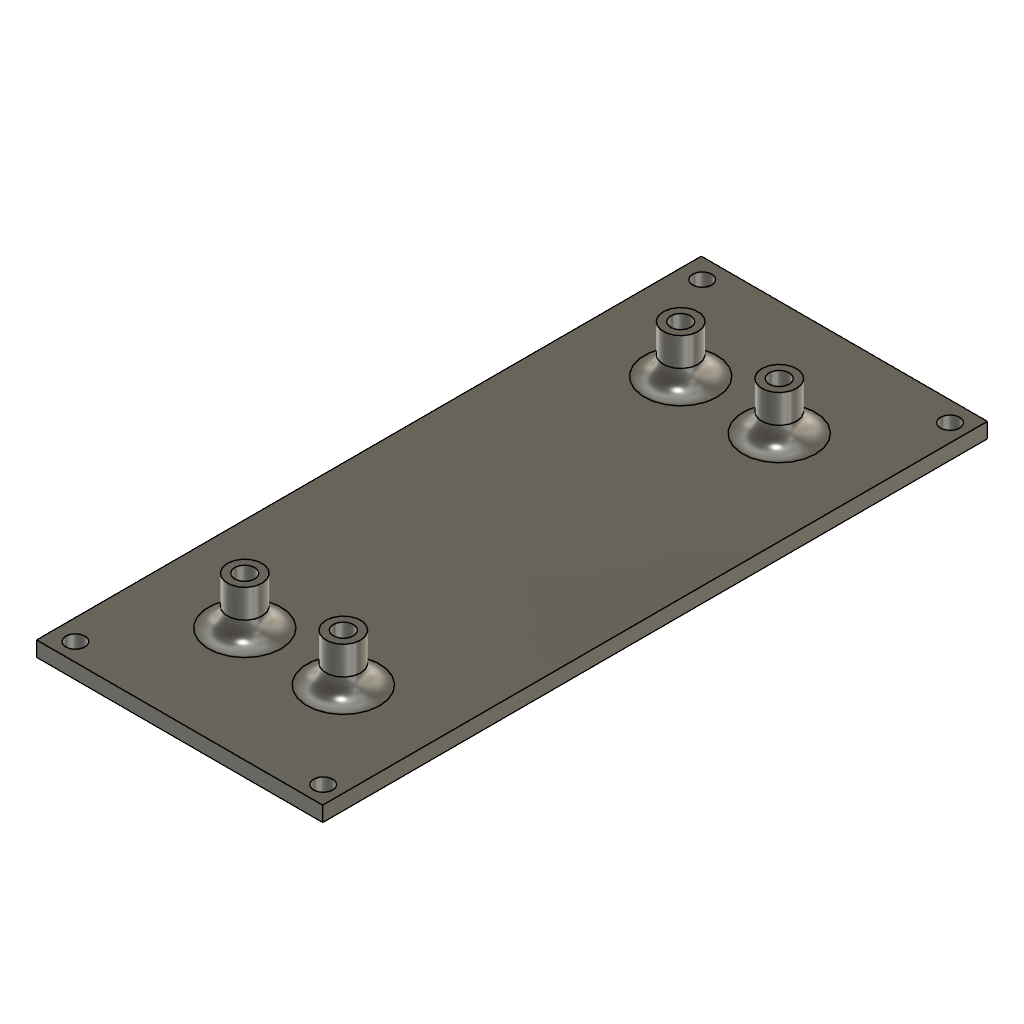
raspberry_pi_pico_mounting_board (Autodesk Fusion 360 design; units mm, degrees)
Autodesk Fusion 360 part; units mm, degrees
sketch "Sketch1" plane through (0, 0, 0) normal (0, 0, 1) x (1, 0, 0)
  line L0 (0, 0) -> (30.2, 0)
  line L1 (30.2, 0) -> (30.2, 70.15)
  line L2 (30.2, 70.15) -> (0, 70.15)
  line L3 (0, 70.15) -> (0, 0)
  dimension "d1" = 30.2
  dimension "d2" = 70.15
  constraint horizontal L0
  constraint vertical L1
  constraint horizontal L2
  constraint vertical L3
  constraint coincident L0.start L3.end
  measures "d1" distance of L0.start L0.end
  measures "d2" distance of L0.start L2.end
extrude "Extrude1" add sketch "Sketch1" along normal blind 1.6
sketch "Sketch3" plane through (0, 0, 1.6) normal (0, 0, 1) x (-1, 0, 0)
  line L0 (0, -70.15) -> (0, 0)
  line L1 (0, 0) -> (-30.2, 0)
  line L2 (-30.2, 0) -> (-30.2, -70.15)
  line L3 (-30.2, -70.15) -> (0, -70.15)
  circle A0 centre (-2.2, -68.05) radius 1
  circle A1 centre (-28.35, -68.05) radius 1
  circle A2 centre (-2.2, -1.9) radius 1
  circle A3 centre (-28.35, -1.9) radius 1
  dimension "d7" = 2
  dimension "d12" = -26.15
  dimension "d13" = 66.15
  dimension "d16" = 2.2
  dimension "d17" = 2.1
  measures "d7" diameter of A0
  measures "d16" distance of L0 A0.centre
  measures "d17" distance of L3 A0.centre
extrude "Extrude2" cut sketch "Sketch3" against normal blind 1.6 contours A0 | A1 | A2 | A3
sketch "Sketch5" plane through (0, 0, 1.6) normal (0, 0, 1) x (-1, 0, 0)
  circle A0 centre (-2.2, -1.9) radius 1
  circle A1 centre (-28.35, -68.05) radius 1
  circle A2 centre (-28.35, -1.9) radius 1
  circle A3 centre (-2.2, -68.05) radius 1
  line L0 (0, -70.15) -> (0, 0)
  line L1 (0, 0) -> (-30.2, 0)
  line L2 (-30.2, 0) -> (-30.2, -70.15)
  line L3 (-30.2, -70.15) -> (0, -70.15)
  line L4 (-9.9, -58.075) -> (-20.3, -58.075) construction
  line L5 (-20.3, -58.075) -> (-20.3, -12.075) construction
  line L6 (-20.3, -12.075) -> (-9.9, -12.075) construction
  line L7 (-9.9, -12.075) -> (-9.9, -58.075) construction
  line L8 (-15.1, -70.15) -> (-15.1, 0) construction
  line L9 (0, -35.075) -> (-30.2, -35.075) construction
  line L10 (-9.9, -35.075) -> (-20.3, -35.075) construction
  line L11 (-15.1, -58.075) -> (-15.1, -12.075) construction
  circle A4 centre (-9.9, -58.075) radius 1.05
  circle A5 centre (-20.3, -58.075) radius 1.05
  circle A6 centre (-9.9, -12.075) radius 1.05
  circle A7 centre (-20.3, -12.075) radius 1.05
  dimension "d18" = 46
  dimension "d19" = 10.4
  dimension "d20" = 2.1
  dimension "d23" = -10.4
  dimension "d24" = 46
  constraint horizontal L4
  constraint vertical L5
  constraint horizontal L6
  constraint vertical L7
  constraint midpoint L3 L8.start
  constraint midpoint L1 L8.end
  constraint midpoint L0 L9.start
  constraint midpoint L2 L9.end
  constraint midpoint L7 L10.start
  constraint midpoint L5 L10.end
  constraint midpoint L4 L11.start
  constraint midpoint L6 L11.end
  constraint coincident L8 L11.start
  constraint coincident L9 L10.start
  constraint coincident L4.start L7.end
  measures "d18" distance of L4.start L6.end
  measures "d19" distance of L4.start L4.end
  measures "d20" diameter of A4
extrude "Extrude3" cut sketch "Sketch5" against normal up to surface (1.6 mm away) contours A4 | A5 | A6 | A7
sketch "Sketch6" plane through (0, 0, 1.6) normal (0, 0, 1) x (-1, 0, 0)
  line L0 (0, -70.15) -> (0, 0)
  line L1 (0, 0) -> (-30.2, 0)
  line L2 (-30.2, 0) -> (-30.2, -70.15)
  line L3 (-30.2, -70.15) -> (0, -70.15)
  circle A0 centre (-2.2, -68.05) radius 1
  circle A1 centre (-28.35, -1.9) radius 1
  circle A2 centre (-28.35, -68.05) radius 1
  circle A3 centre (-2.2, -1.9) radius 1
  circle A4 centre (-9.9, -58.075) radius 1.05
  circle A5 centre (-20.3, -12.075) radius 1.05
  circle A6 centre (-20.3, -58.075) radius 1.05
  circle A7 centre (-9.9, -12.075) radius 1.05
  circle A8 centre (-9.9, -58.075) radius 1.05
  circle A9 centre (-9.9, -58.075) radius 1.825
  circle A10 centre (-20.3, -58.075) radius 1.825
  circle A11 centre (-20.3, -58.075) radius 1.05
  circle A12 centre (-9.9, -12.075) radius 1.825
  circle A13 centre (-9.9, -12.075) radius 1.05
  circle A14 centre (-20.3, -12.075) radius 1.825
  circle A15 centre (-20.3, -12.075) radius 1.05
  dimension "d27" = 3.65
  dimension "d28" = 2.1
  dimension "d31" = -10.4
  dimension "d32" = 46
  constraint concentric A4 A8
  constraint concentric A4 A9
  measures "d27" diameter of A9
  measures "d28" diameter of A8
extrude "Extrude4" add sketch "Sketch6" along normal blind 5 contours A9 | A10 | A12 | A14
fillet "Fillet1" radius 2 4 edges at (22.0015, 11.4151, 1.6) (11.6015, 11.4151, 1.6) (11.6015, 57.4151, 1.6) (22.0015, 57.4151, 1.6)
